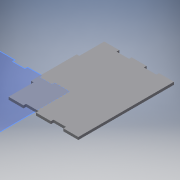
# Autodesk Inventor part: Base Plate
Saved by Autodesk Inventor 2016 (Build 200138000, 138)
## iProperties
Created: 2016-11-04
Part Number: Base Plate
Material: Generic
Document SubType Name: Modeling
Designer: william
Density: 1 g/cm^3
Appearance: Default
Author: william
Autodesk Inventor part; units mm, degrees
ref_plane "YZ Plane" through (0, 0, 0) normal (1, 0, 0) x (0, 1, 0)
ref_plane "XZ Plane" through (0, 0, 0) normal (0, 1, 0) x (-1, 0, 0)
ref_plane "XY Plane" through (0, 0, 0) normal (0, 0, 1) x (1, 0, 0)
sketch "Sketch1" plane through (0, 0, 0) normal (0, 0, 1) x (1, 0, 0)
  line L0 (0, 0) -> (145.2, 0)
  line L1 (145.2, 0) -> (145.2, 192)
  line L2 (145.2, 192) -> (0, 192)
  line L3 (0, 192) -> (0, 0)
  line L4 (145.2, 192) -> (110.498, 192)
  line L5 (145.2, 186.8) -> (145.2, 192)
  line L6 (85.92, 192) -> (45.5217, 192)
  line L7 (21.953, 192) -> (0, 192)
  line L8 (0, 192) -> (0, 185.7065)
  line L9 (35.2, 192) -> (60.2, 192)
  line L10 (60.2, 192) -> (60.2, 186.8)
  line L11 (60.2, 186.8) -> (35.2, 186.8)
  line L12 (35.2, 186.8) -> (35.2, 192)
  line L13 (90.2, 192) -> (115.2, 192)
  line L14 (115.2, 192) -> (115.2, 186.8)
  line L15 (115.2, 186.8) -> (90.2, 186.8)
  line L16 (90.2, 186.8) -> (90.2, 192)
  line L17 (0, 192) -> (5.2, 192)
  line L18 (5.2, 192) -> (5.2, 142)
  line L19 (5.2, 142) -> (0, 142)
  line L20 (0, 142) -> (0, 192)
  line L21 (0, 96) -> (145.2, 96) construction
  line L22 (0, 0) -> (5.2, 0)
  line L23 (5.2, 0) -> (5.2, 50)
  line L24 (5.2, 50) -> (0, 50)
  line L25 (0, 50) -> (0, 0)
  line L26 (35.2, 0) -> (60.2, 0)
  line L27 (60.2, 0) -> (60.2, 5.2)
  line L28 (60.2, 5.2) -> (35.2, 5.2)
  line L29 (35.2, 5.2) -> (35.2, 0)
  line L30 (90.2, 0) -> (115.2, 0)
  line L31 (115.2, 0) -> (115.2, 5.2)
  line L32 (115.2, 5.2) -> (90.2, 5.2)
  line L33 (90.2, 5.2) -> (90.2, 0)
  dimension "d0" = 192
  dimension "d1" = 145.2
  dimension "d6" = 25
  dimension "d7" = 25
  dimension "d8" = 5.2
  dimension "d9" = 30
  dimension "d10" = 30
  dimension "d11" = 50
  dimension "d12" = 5.2
  dimension "d13" = 50
  dimension "d14" = 5.2
  dimension "d15" = 25
  dimension "d16" = 25
  dimension "d17" = 5.2
  dimension "d18" = 30
  dimension "d19" = 30
  constraints: 68 end point, 14 parallel, 10 horizontal, 9 point on line, 8 perpendicular, 2 midpoint
  measures "d0" distance of L0.end L1.end
  measures "d1" distance of L1.end L2.end
  measures "d6" distance of L10.end L11.end
  measures "d7" distance of L14.end L15.end
  measures "d8" distance of L9.end L10.end
  measures "d9" distance between parallel lines of L1 L14
  measures "d10" distance between parallel lines of L16 L10
  measures "d11" distance of L17.end L18.end
  measures "d12" distance of L18.end L19.end
  measures "d13" distance of L22.end L23.end
  measures "d14" distance of L23.end L24.end
  measures "d15" distance of L27.end L28.end
  measures "d16" distance of L31.end L32.end
  measures "d17" distance of L26.end L27.end
  measures "d18" distance between parallel lines of L1 L31
  measures "d19" distance between parallel lines of L33 L27
extrude "Extrusion2" add sketch "Sketch1" along normal blind 5.2 contours L23 L24 L3 L19 L18 L2 L12 L11 L10 L16 L15 L14 L1 L0 L31 L32 L33 L27 L28 L29
body "Solid2"
